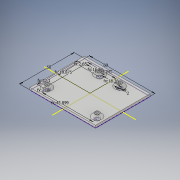
# Autodesk Inventor part: Panel mount plate
Saved by Autodesk Inventor 2018.3 (Build 223284000, 284)
## iProperties
Created: 2020-05-25
Part Number: Panel mount plate
Material: Generic
Document SubType Name: Modeling
Designer: uqspowe6
Density: 1 g/cm^3
Appearance: Default
Author: uqspowe6
Autodesk Inventor part; units mm, degrees
ref_plane "YZ Plane" through (0, 0, 0) normal (1, 0, 0) x (0, 1, 0)
ref_plane "XZ Plane" through (0, 0, 0) normal (0, 1, 0) x (-1, 0, 0)
ref_plane "XY Plane" through (0, 0, 0) normal (0, 0, 1) x (1, 0, 0)
sketch "Sketch1" plane through (0, 0, 0) normal (0, 1, 0) x (-1, 0, 0)
  circle A0 centre (-9.9449, -17.225) radius 1 construction
  circle A1 centre (8.4149, -17.225) radius 1 construction
  circle A2 centre (22.1847, 17.225) radius 1 construction
  circle A3 centre (-23.7147, 17.225) radius 1 construction
  circle A4 centre (-9.9449, -17.225) radius 2
  circle A5 centre (8.4149, -17.225) radius 2
  circle A6 centre (22.1847, 17.225) radius 2
  circle A7 centre (-23.7147, 17.225) radius 2
  line L0 (30, -25) -> (-30, -25)
  line L1 (-30, -25) -> (-30, 25)
  line L2 (-30, 25) -> (30, 25)
  line L3 (30, 25) -> (30, -25)
  line L4 (0, -35) -> (0, 35) projected
  line L5 (42, 0) -> (-42, 0) projected
  point P0 (0, 0)
  point P1 (25.2446, -19.875)
  dimension "d0" = 25.2446
  dimension "d1" = 19.875
  dimension "d2" = 16.8298
  dimension "d3" = 18.3597
  dimension "d4" = 2.65
  dimension "d5" = 37.1
  dimension "d6" = 3.06
  dimension "d7" = 45.8993
  dimension "d9" = 2
  dimension "d10" = 1
  dimension "d11" = 60
  dimension "d12" = 50
  constraints: 8 centre point, 8 coincident, 8 end point, 6 equal radius, 2 horizontal alignment, 2 parallel, 1 horizontal, 1 perpendicular, 2 other
  measures "d0" horizontal distance of point (0, 0) point (25.245, -19.875)
  measures "d1" vertical distance of point (0, 0) point (25.245, -19.875)
  measures "d2" horizontal distance of point (8.415, -17.225) point (25.245, -19.875)
  measures "d3" distance of point (-9.945, -17.225) point (8.415, -17.225)
  measures "d4" vertical distance of point (8.415, -17.225) point (25.245, -19.875)
  measures "d5" vertical distance of point (22.185, 17.225) point (25.245, -19.875)
  measures "d6" horizontal distance of point (22.185, 17.225) point (25.245, -19.875)
  measures "d7" distance of point (-23.715, 17.225) point (22.185, 17.225)
  measures "d9" diameter of A0
  measures "d10" radial gap between concentric circles of A4 A0
  measures "d11" distance of L0.start L0.end
  measures "d12" distance of L2.end L0.start
extrude "Extrusion1" add sketch "Sketch1" along normal blind 5 contours A4 | A5 | A6 | A7
extrude "Extrusion2" add sketch "Sketch1" along normal blind 2
chamfer "Chamfer1" distance 2.5 angle 45 4 edges at (-6.4149, 2, -17.225) (11.9449, 2, -17.225) (25.7147, 2, 17.225) (-20.1847, 2, 17.225)
hole "Hole1" at (-8.4149, 0, -17.225) at (9.9449, 0, -17.225) at (-22.1847, 0, 17.225) at (23.7147, 0, 17.225) direction (0, 1, 0) diameter 2.2 end through all counterbore diameter 4.4 counterbore depth 1.6 clearance for "Hex Head Machine Screw" size "M2" standard "Ansi Metric M Profile"
equation "\"d0\" = origin_x"
equation "\"d1\" = origin_y"
equation "\"d2\" = 3 * pitch_x + 0.5 * cell_w"
equation "\"d3\" = 4 * pitch_x"
equation "\"d4\" = 0.5 * pitch"
equation "\"d5\" = 7 * pitch"
equation "\"d6\" = 0.5 * cell_w"
equation "\"d7\" = 10 * pitch_x"
equation "\"pitch\" = 5.3"
equation "\"pitch_x\" = 0.866025 * pitch"
equation "\"cell_w\" = 1.1547 * pitch"
equation "\"origin_x\" = 25.244641"
equation "\"origin_y\" = 19.875"
body "Solid1"
